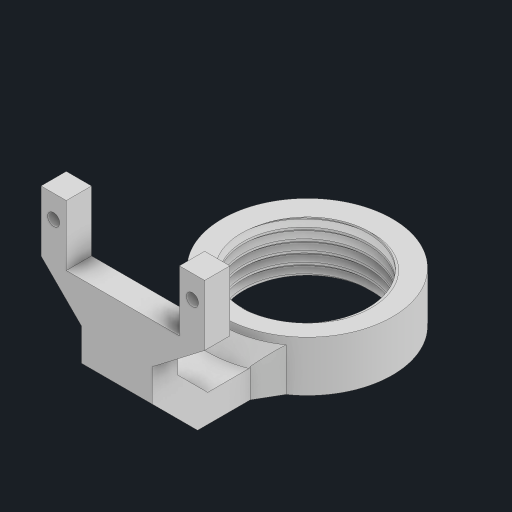
# Autodesk Inventor part: TH_acople_servo_valvula
Saved by Autodesk Inventor 2024.1 (Build 281209000, 209)
## iProperties
Created: 2024-11-06
Part Number: TH_acople_servo_valvula
Material: Generic
Document SubType Name: Modeling
Designer: luisg
Density: 1 g/cm^3
Appearance: Default
Author: luisg
Autodesk Inventor part; units mm, degrees
ref_plane "YZ Plane" through (0, 0, 0) normal (1, 0, 0) x (0, 1, 0)
ref_plane "XZ Plane" through (0, 0, 0) normal (0, 1, 0) x (-1, 0, 0)
sketch "Sketch1" plane through (0, 0, 0) normal (0, 1, 0) x (-1, 0, 0)
  circle A0 centre (0, 0) radius 12.3325
  circle A1 centre (0, 0) radius 16.8325
  dimension "d0" = 24.5
  dimension "d1" = 4.5
  constraints: 2 centre point, 1 coincident
  measures "d1" radial gap between concentric circles of A0 A1
extrude "Extrusion1" add sketch "Sketch1" along normal blind 10
sketch "Sketch2" plane through (0, 0, 0) normal (1, 0, 0) x (0, 1, 0)
  line L0 (13.5671, -12.3325) -> (12.9435, -13.4125)
  line L1 (12.9435, -13.4125) -> (12.6235, -13.4125)
  line L2 (12.6235, -13.4125) -> (12, -12.3325)
  line L3 (12, -12.3325) -> (13.5671, -12.3325)
  line L4 (10, -12.3325) -> (0, -12.3325) construction
  point P0 (0, 0)
  dimension "d4" = 60
  dimension "d5" = 0.25
  dimension "d6" = 1.08
  dimension "d7" = 2
  constraints: 8 end point, 2 horizontal, 1 collinear, 1 equal length
  measures "d4" angle of L2 L0
  measures "d6" distance between parallel lines of L3 L1
  measures "d7" distance of L4.start L2.end
coil "Coil1" sketch "Sketch2" operation cut axis through (0, -10, 0) along (0, -1, 0) pitch 2 turns 10 hand right
ref_plane "Work Plane4" through (0, 0, 37.7325) normal (0, 0, 1) x (1, 0, 0)
ref_plane "Work Plane3" through (0, 0, 16.8325) normal (0, 0, 1) x (1, 0, 0)
sketch "Sketch6" plane through (0, 0, 37.7325) normal (0, 0, 1) x (1, 0, 0)
  line L0 (-7, 0) -> (-7, 15.4)
  line L1 (-7, 15.4) -> (-15, 23.4)
  line L2 (-15, 23.4) -> (-15, 35.4)
  line L3 (-15, 35.4) -> (17.4, 35.4)
  line L4 (17.4, 35.4) -> (17.4, 23.4)
  line L5 (17.4, 23.4) -> (7, 15.4)
  line L6 (7, 15.4) -> (7, 0)
  line L7 (7, 0) -> (-7, 0)
  line L8 (-10, 35.4) -> (-10, 23.4)
  line L9 (-10, 23.4) -> (12.4, 23.4)
  line L10 (12.4, 23.4) -> (12.4, 35.4)
  point P0 (0, 0)
  point P1 (0, 0)
  point P2 (-15, 29.4)
  dimension "d31" = 14
  dimension "d32" = 15.4
  dimension "d33" = 135
  dimension "d37" = 12
  dimension "d38" = 8
  dimension "d39" = 17.4
  dimension "d40" = 5
  dimension "d41" = 5
  dimension "d43" = 12
  dimension "d45" = 10
  dimension "d47" = 22.4
  constraints: 22 end point, 4 perpendicular, 2 horizontal, 2 midpoint, 2 parallel, 2 point on line, 1 coincident
  measures "d31" distance of L6.end L0.start
  measures "d32" distance of L5.end L6.end
  measures "d33" angle of L0 L1
  measures "d37" distance of L1.end L2.end
  measures "d38" vertical distance of L5.end L4.end
  measures "d39" horizontal distance of L4.end point (0, 0)
  measures "d40" distance between parallel lines of L8 L2
  measures "d41" distance between parallel lines of L4 L10
  measures "d43" distance between parallel lines of L9 L3
  measures "d45" distance from line of L8 point (0, 0)
  measures "d47" distance between parallel lines of L10 L8
extrude "Extrusion4" add sketch "Sketch6" against normal blind 5 contours L0 L1 L2 L3 L8 L9 L10 L4 L5 L6 L7
sketch "Sketch7" plane through (0, 0, 0) normal (0, 1, 0) x (-1, 0, 0)
  line L0 (-7, 32.7325) -> (7, 32.7325) projected
  circle A0 centre (0, 0) radius 16.8325 projected
  line L1 (-7, 32.7325) -> (-7, 15.3079)
  line L2 (7, 32.7325) -> (7, 15.3079)
  constraints: 4 end point, 2 point on circle, 2 vertical
extrude "Extrusion5" add sketch "Sketch7" along normal blind 5.5 contours L0 L2 A0 L1
chamfer "Chamfer2" distance 6 angle 45 1 edges at (0, 5.5, 32.7325)
chamfer "Chamfer3" distance 9 angle 45 1 edges at (0, 0, 37.7325)
sketch "Sketch8" plane through (0, 0, 37.7325) normal (0, 0, 1) x (1, 0, 0)
  line L0 (-10, 35.4) -> (-15, 35.4) projected
  line L1 (17.4, 35.4) -> (12.4, 35.4) projected
  circle A0 centre (-12.5, 30.8964) radius 1.185
  circle A1 centre (14.9782, 30.8964) radius 1.185
  point P0 (0, 0)
  point P1 (-12.5, 35.4)
  dimension "d58" = 2.3
  constraints: 2 centre point, 1 equal radius, 1 horizontal alignment, 1 midpoint, 1 vertical alignment
extrude "Extrusion6" cut sketch "Sketch8" against normal through all
chamfer "Chamfer4" distance 3 angle 45 1 edges at (0, 5.5, 16.8325)
chamfer "Chamfer5" distance 3 angle 45 4 edges at (-7, 7, 15.3079) (-7, 2.75, 15.3079) (7, 7, 15.3079) (7, 2.75, 15.3079)
body "Solid1"
